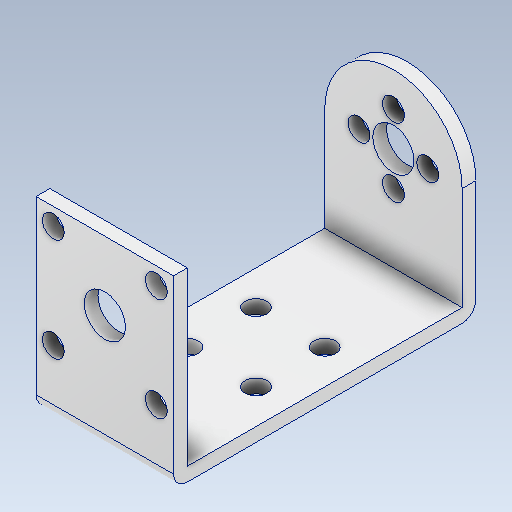
# Autodesk Inventor part: サーボモーター25kgcmサーボホーン3
Saved by Autodesk Inventor 2021 (Build 250183000, 183)
## iProperties
Created: 2020-02-02
Part Number: サーボモーター25kgcmサーボホーン3
Material: アルミニウム 6061
Document SubType Name: Modeling
Designer: yuta2
Density: 2.7 g/cm^3
Appearance: アルミニウム - フラット
Mass: 9.00101 g
Surface Area: 40.8578 cm^2
Volume: 3.33371 cm^3
Author: yuta2
Autodesk Inventor part; units mm, degrees
ref_plane "YZ Plane" through (0, 0, 0) normal (1, 0, 0) x (0, 1, 0)
ref_plane "XZ Plane" through (0, 0, 0) normal (0, 1, 0) x (-1, 0, 0)
ref_plane "XY Plane" through (0, 0, 0) normal (0, 0, 1) x (1, 0, 0)
sketch "スケッチ1" plane through (0, 0, 0) normal (1, 0, 0) x (0, 1, 0)
  line L0 (0, 0) -> (-2, 0)
  line L1 (-2, 0) -> (-2, -44)
  line L2 (-2, -44) -> (0, -44)
  line L3 (0, -44) -> (0, 0)
  line L4 (0, -44) -> (25, -44)
  line L5 (25, -44) -> (25, -42)
  line L6 (25, -42) -> (0, -42)
  line L7 (0, -42) -> (0, -44)
  line L8 (0, 0) -> (25, 0)
  line L9 (25, 0) -> (25, -2)
  line L10 (25, -2) -> (0, -2)
  line L11 (0, -2) -> (0, 0)
  dimension "d0" = 2
  dimension "d1" = 44
  dimension "d2" = 25
  dimension "d3" = 2
  dimension "d4" = 25
  dimension "d5" = 2
  constraints: 24 end point, 6 parallel, 3 horizontal, 3 perpendicular
  measures "d0" distance of L2.end L1.end
  measures "d1" distance of L1.end L0.end
  measures "d2" distance of L6.end L5.end
  measures "d3" distance of L5.end L4.end
  measures "d4" distance of L9.end L10.end
  measures "d5" distance of L8.end L9.end
extrude "押し出し1" add sketch "スケッチ1" along normal blind 20
sketch "スケッチ2" plane through (0, -2, 0) normal (0, 0, 1) x (1, 0, 0)
  line L0 (0, 27) -> (0, 0) projected
  line L1 (0, 27) -> (20, 27) projected
  point P0 (0, 2)
  point P1 (2.5, 24.5)
  point P2 (17.5, 24.5)
  point P3 (17.5, 9.5)
  point P4 (2.5, 9.5)
  dimension "d8" = 2.5
  dimension "d9" = 15
  dimension "d10" = 15
  dimension "d11" = 17.5
  constraints: 2 horizontal alignment, 2 vertical alignment
  measures "d8" distance from line of L0 point (2.5, 9.5)
  measures "d9" distance of point (17.5, 9.5) point (2.5, 9.5)
  measures "d10" distance of point (2.5, 9.5) point (2.5, 24.5)
  measures "d11" distance from line of L1 point (2.5, 9.5)
hole "穴1" at (2.5, 22.5, 0) at (17.5, 22.5, 0) at (17.5, 7.5, 0) at (2.5, 7.5, 0) direction (0, 0, -1) diameter 3.2 depth 2 tip angle 118
sketch "スケッチ3" plane through (0, -2, 0) normal (0, 0, 1) x (1, 0, 0)
  circle A0 centre (10, 17) radius 3
  line L0 (0, 27) -> (20, 27) projected
  line L1 (0, 27) -> (0, 0) projected
  point P0 (0, 2)
  dimension "d19" = 6
  dimension "d20" = 10
  dimension "d21" = 10
  constraints: 1 centre point
  measures "d19" diameter of A0
  measures "d20" distance from line of L0 A0.centre
  measures "d21" distance from line of L1 A0.centre
extrude "押し出し2" cut sketch "スケッチ3" against normal through all
sketch "スケッチ4" plane through (0, -2, -44) normal (0, 0, -1) x (-1, 0, 0)
  circle A0 centre (-10, 17) radius 3 projected
  circle A1 centre (-10, 17) radius 5
  point P0 (0, 2)
  point P1 (-10, 22)
  point P2 (-15, 17)
  point P3 (-5, 17)
  point P4 (-10, 12)
  dimension "d24" = 10
  constraints: 4 point on circle, 2 horizontal alignment, 2 vertical alignment, 1 centre point, 1 coincident
  measures "d24" diameter of A1
hole "穴2" at (10, 20, -44) at (15, 15, -44) at (5, 15, -44) at (10, 10, -44) direction (0, 0, 1) diameter 3.2 depth 2 tip angle 118
sketch "スケッチ5" plane through (0, -2, -44) normal (0, 0, -1) x (-1, 0, 0)
  circle A0 centre (-10, 17) radius 3 projected
  circle A1 centre (-10, 17) radius 10
  line L0 (-20, 27) -> (-20, 2) projected
  line L1 (-20, 17) -> (0, 17)
  line L2 (0, 17) -> (0, 27)
  line L3 (0, 27) -> (-20, 27)
  line L4 (-20, 27) -> (-20, 17)
  point P0 (0, 2)
  point P1 (-10, 27)
  dimension "d32" = 20
  constraints: 8 end point, 2 parallel, 1 coincident, 1 horizontal, 1 perpendicular, 1 point on line, 3 other
extrude "押し出し3" cut sketch "スケッチ5" against normal blind 2 contours A1 L3 L2 | L0 L3 A1
sketch "スケッチ6" plane through (0, -2, -44) normal (0, -1, 0) x (1, 0, 0)
  line L0 (11.6, 0) -> (8.4, 0) projected
  line L1 (10, 0) -> (10, 44)
  line L2 (7, 44) -> (13, 44) projected
  line L3 (0, 2) -> (0, 42) projected
  line L4 (0, 22) -> (20, 22)
  line L5 (20, 2) -> (20, 42) projected
  point P0 (0, 44)
  point P1 (5, 17)
  point P2 (5, 27)
  point P3 (15, 27)
  point P4 (15, 17)
  dimension "d35" = 10
  dimension "d36" = 10
  constraints: 4 end point, 4 midpoint, 3 symmetric about line
  measures "d35" distance of point (15, 17) point (5, 17)
  measures "d36" distance of point (15, 27) point (15, 17)
hole "穴3" at (5, -2, -27) at (5, -2, -17) at (15, -2, -17) at (15, -2, -27) direction (0, 1, 0) diameter 3.2 depth 2 tip angle 118
fillet "フィレット1" radius 2 2 edges at (10, -2, -44) (10, -2, 0)
